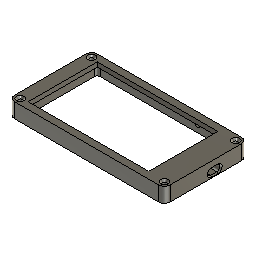
inky-ical (Autodesk Fusion 360 design; units mm, degrees)
Autodesk Fusion 360 part; units mm, degrees
note: some values were not read from the file. Set by a fixed rule: which face or edge a step refers to.
sketch "base" plane through (0, 0, 0) normal (0, 0, 1) x (1, 0, 0)
  line L0 (-5, 62.75) -> (-5, 0)
  line L1 (0, -5) -> (126.75, -5)
  line L2 (0, 67.75) -> (126.75, 67.75)
  line L3 (131.75, 62.75) -> (131.75, 0)
  arc A0 (0, 67.75) -> (-5, 62.75) centre (0, 62.75) ccw
  arc A1 (131.75, 62.75) -> (126.75, 67.75) centre (126.75, 62.75) ccw
  arc A2 (126.75, -5) -> (131.75, 0) centre (126.75, 0) ccw
  arc A3 (-5, 0) -> (0, -5) centre (0, 0) ccw
  line L4 (8, 59.75) -> (110, 59.75)
  line L5 (110, 59.75) -> (110, 3)
  line L6 (110, 3) -> (8, 3)
  line L7 (8, 3) -> (8, 59.75)
  line L8 (3, 64.75) -> (123.75, 64.75)
  line L9 (123.75, 64.75) -> (123.75, -2)
  line L10 (123.75, -2) -> (3, -2)
  line L11 (3, -2) -> (3, 64.75)
  line L12 (3, -2) -> (8, 3) construction
  line L13 (3, 64.75) -> (8, 59.75) construction
  circle A4 centre (0, 62.75) radius 1.75
  circle A5 centre (0, 0) radius 1.75
  circle A6 centre (126.75, 0) radius 1.75
  circle A7 centre (126.75, 62.75) radius 1.75
  dimension "outerCornerRadius" = 5
  dimension "d2" = 5
  dimension "d3" = 5
  dimension "d4" = 5
  dimension "d5" = 102
  dimension "d6" = 56.75
  dimension "d7" = 120.75
  dimension "d8" = 66.75
  dimension "d10" = 3
  dimension "d11" = 3
  dimension "m3ScrewHole" = 3.5
  dimension "d14" = 3.5
  dimension "d15" = 3.5
  dimension "d16" = 3.5
  dimension "d18" = 3
  dimension "d19" = 3
  dimension "d40" = 5
  constraint vertical L0
  constraint horizontal L1
  constraint horizontal L2
  constraint vertical L3
  constraint tangent L0 A0
  constraint tangent L2 A1
  constraint tangent L1 A2
  constraint tangent L1 A3
  constraint tangent L2 A0
  constraint tangent L3 A1
  constraint tangent L3 A2
  constraint tangent L0 A3
  constraint horizontal L4
  constraint vertical L5
  constraint horizontal L6
  constraint vertical L7
  constraint coincident A3.centre A5.centre
  constraint horizontal L8
  constraint vertical L9
  constraint horizontal L10
  constraint vertical L11
  constraint equal L12 L13
  constraint concentric A0 A4
  constraint concentric A2 A6
  constraint concentric A1 A7
  measures "outerCornerRadius" radius of A3
  measures "d2" radius of A0
  measures "d3" radius of A1
  measures "d4" radius of A2
  measures "d5" distance of L5.end L6.end
  measures "d6" distance of L4.end L5.end
  measures "d7" distance of L9.end L10.end
  measures "d8" distance of L8.end L9.end
  measures "d10" distance of L1 L10
  measures "d11" distance of L2 L8
  measures "m3ScrewHole" diameter of A4
  measures "d14" diameter of A5
  measures "d15" diameter of A6
  measures "d16" diameter of A7
  measures "d18" distance of L11 A0.centre
  measures "d19" distance of A1.centre L9
  measures "d40" distance of L7 L11
  measures "d45" diameter of L3.end
  measures "d53" distance of L3.end
  measures "d59" diameter of L3.end
  measures "d60" diameter of L3.end
extrude "Extrude1" add sketch "base" along normal blind 13 contours L0 L1 L2 L3 A0 A1 A2 A3 | L8 L9 L10 L11 makes body 1
chamfer "Chamfer1" distance 1.6 angle 45 4 edges at (-1.6316, 0.6328, 13) (-1.6316, 63.3828, 13) (125.1184, 63.3828, 13) (125.1184, 0.6328, 13) tangent chain off on bodies 1
extrude "Extrude2" cut sketch "base" along normal blind 11 contours L8 L9 L10 L11 bodies 1
chamfer "Chamfer3" distance 2 angle 45 4 edges at (59, 3, 13) (110, 31.375, 13) (8, 31.375, 13) (59, 59.75, 13) tangent chain off on bodies 1
extrude "Extrude3" add sketch "base" against normal blind 8.5 separate body contours L0 L1 L2 L3 A0 A1 A2 A3 | L4 L5 L6 L7 | L8 L9 L10 L11 | A4 | A5 | A6 | A7 makes body 2
sketch "battery-magnet-recess" plane through (0, 0, 0) normal (0, 0, 1) x (-1, 0, 0)
  arc A0 (0, -67.75) -> (5, -62.75) centre (0, -62.75) ccw
  line L0 (5, -62.75) -> (5, 0)
  arc A1 (5, 0) -> (0, 5) centre (0, 0) ccw
  line L1 (0, 5) -> (-126.75, 5)
  arc A2 (-126.75, 5) -> (-131.75, 0) centre (-126.75, 0) ccw
  line L2 (-131.75, 0) -> (-131.75, -62.75)
  arc A3 (-131.75, -62.75) -> (-126.75, -67.75) centre (-126.75, -62.75) ccw
  line L3 (-126.75, -67.75) -> (0, -67.75)
  line L4 (-109.75, -0.875) -> (-15.75, -0.875)
  line L5 (-15.75, -0.875) -> (-15.75, -61.875)
  line L6 (-15.75, -61.875) -> (-109.75, -61.875)
  line L7 (-109.75, -61.875) -> (-109.75, -0.875)
  line L8 (-3, 2) -> (-3, -64.75)
  line L9 (-123.75, 2) -> (-3, 2)
  circle A4 centre (-126.75, 0) radius 2.25
  circle A5 centre (-126.75, -62.75) radius 2.25
  circle A6 centre (0, -62.75) radius 2.25
  circle A7 centre (0, 0) radius 2.25
  line L10 (-109.75, -31.375) -> (-131.75, -31.375) construction
  circle A8 centre (-3, -9.375) radius 4.1
  circle A9 centre (-3, -53.375) radius 4.1
  circle A10 centre (-123.75, -53.375) radius 4.1
  circle A11 centre (-123.75, -9.375) radius 4.1
  line L11 (-3, -53.375) -> (-3, -9.375) construction
  line L12 (-123.75, -53.375) -> (-123.75, -9.375) construction
  line L13 (5, -31.375) -> (-3, -31.375) construction
  line L14 (-123.75, -31.375) -> (-131.75, -31.375) construction
  dimension "d29" = 61
  dimension "d30" = 94
  dimension "d33" = 4.5
  dimension "d53" = 22
  dimension "d57" = 8.2
  dimension "d58" = 8.2
  dimension "d59" = 8.2
  dimension "d60" = 8.2
  dimension "d64" = 8
  dimension "d65" = 44
  dimension "d66" = 8
  constraint horizontal L4
  constraint vertical L5
  constraint horizontal L6
  constraint vertical L7
  constraint concentric A2 A4
  constraint concentric A3 A5
  constraint concentric A0 A6
  constraint concentric A1 A7
  constraint equal A4 A7
  constraint equal A4 A6
  constraint equal A4 A5
  constraint coincident L7 L10.start
  constraint coincident L2 L10.end
  constraint perpendicular L2 L10
  constraint midpoint L2 L10.end
  constraint midpoint L7 L10.start
  constraint coincident A9.centre L11.start
  constraint coincident A8.centre L11.end
  constraint coincident A10.centre L12.start
  constraint coincident A11.centre L12.end
  constraint vertical L11
  constraint vertical L12
  constraint coincident L0 L13.start
  constraint coincident L11 L13.end
  constraint perpendicular L11 L13
  constraint midpoint L11 L13.end
  constraint midpoint L0 L13.start
  constraint equal L11 L12
  constraint coincident L12 L14.start
  constraint perpendicular L2 L14
  constraint midpoint L12 L14.start
  measures "d29" distance of L4.start L6.end
  measures "d30" distance of L5.end L6.end
  measures "d33" diameter of A4
  measures "d53" distance of L10.start L10.end
  measures "d57" diameter of A8
  measures "d58" diameter of A9
  measures "d59" diameter of A10
  measures "d60" diameter of A11
  measures "d64" distance of L13.start L13.end
  measures "d65" distance of A9.centre A8.centre
  measures "d66" distance of L14.start L10.end
extrude "Extrude4" cut sketch "battery-magnet-recess" against normal blind 6.5 contours L4 L5 L6 L7 bodies 2
extrude "Extrude5" cut sketch "battery-magnet-recess" against normal blind 19 contours A4 | A5 | A6 | A7 bodies 2
fillet "Fillet1" radius 2.5 4 edges at (123.75, 64.75, 5.5) (3, 64.75, 5.5) (3, -2, 5.5) (123.75, -2, 5.5) on bodies 1
fillet "Fillet2" radius 3 2 edges at (62.75, 61.875, -6.5) (62.75, 0.875, -6.5) on bodies 2
sketch "usb-hole" plane through (131.75, 0, 0) normal (1, 0, 0) x (0, 1, 0)
  line L0 (0, 0) -> (62.75, 0)
  line L1 (62.75, 0) -> (62.75, 13)
  line L2 (62.75, 13) -> (0, 13)
  line L3 (0, 13) -> (0, 0)
  line L4 (42, 1.5) -> (36.5, 1.5)
  line L5 (42, 7) -> (36.5, 7)
  arc A0 (42, 1.5) -> (42, 7) centre (42, 4.25) ccw
  arc A1 (36.5, 7) -> (36.5, 1.5) centre (36.5, 4.25) ccw
  line L6 (33.75, 2.1871) -> (33.75, 6.5143) construction
  line L7 (44.75, 2.1572) -> (44.75, 6.4585) construction
  line L8 (62.75, 0) -> (0, 0) construction
  dimension "d41" = 5.5
  dimension "d42" = 11
  dimension "d43" = 1.5
  dimension "d44" = 18
  constraint parallel L2 L4
  constraint parallel L2 L5
  constraint tangent L4 A0
  constraint tangent L4 A1
  constraint equal L4 L5
  constraint tangent L5 A0
  constraint vertical L7
  constraint vertical L6
  constraint tangent A0 L7
  constraint tangent A1 L6
  measures "d41" distance of L4 L5
  measures "d42" distance of L6 L7
  measures "d43" distance of L4 L8
  measures "d44" distance of L1 L7
sketch "reset-button-hole" plane through (0, 67.75, 0) normal (0, 1, 0) x (-1, 0, 0)
  line L0 (-126.75, 0) -> (0, 0)
  line L1 (0, 0) -> (0, 13)
  line L2 (0, 13) -> (-126.75, 13)
  line L3 (-126.75, 13) -> (-126.75, 0)
  circle A0 centre (-91.25, 6.75) radius 2.5
  line L4 (0, 0) -> (-126.75, 0)
  dimension "d45" = 5
  dimension "d46" = 6.75
  dimension "d47" = 35.5
  measures "d45" diameter of A0
  measures "d46" distance of A0.centre L4
  measures "d47" distance of L3 A0.centre
extrude "Extrude6" cut sketch "usb-hole" against normal blind 12 contours L4 L5 A0 A1 bodies 1
extrude "Extrude7" cut sketch "reset-button-hole" against normal blind 7 contours A0 bodies 1
extrude "Extrude9" cut sketch "battery-magnet-recess" against normal blind 8.125 contours L8 A8 | L8 A8 | L8 A9 | L8 A9 | A10 | A11 bodies 2
sketch "mounting-pillars" plane through (0, 0, 0) normal (0, 0, 1) x (-1, 0, 0)
  circle A0 centre (-126.75, 0) radius 2.25
  circle A1 centre (0, 0) radius 2.25
  circle A2 centre (-126.75, -62.75) radius 2.25
  circle A3 centre (0, -62.75) radius 2.25
  arc A4 (0, -67.75) -> (5, -62.75) centre (0, -62.75) ccw
  line L0 (5, -62.75) -> (5, 0)
  arc A5 (5, 0) -> (0, 5) centre (0, 0) ccw
  line L1 (0, 5) -> (-126.75, 5)
  arc A6 (-126.75, 5) -> (-131.75, 0) centre (-126.75, 0) ccw
  line L2 (-131.75, 0) -> (-131.75, -62.75)
  arc A7 (-131.75, -62.75) -> (-126.75, -67.75) centre (-126.75, -62.75) ccw
  line L3 (-126.75, -67.75) -> (0, -67.75)
  line L4 (-109.75, -61.875) -> (-109.75, -0.875)
  line L5 (-109.75, -0.875) -> (-15.75, -0.875)
  line L6 (-15.75, -0.875) -> (-15.75, -61.875)
  line L7 (-15.75, -61.875) -> (-109.75, -61.875)
  circle A8 centre (-123.75, -9.375) radius 4.1
  circle A9 centre (-3, -53.375) radius 4.1
  circle A10 centre (-123.75, -53.375) radius 4.1
  circle A11 centre (-3, -9.375) radius 4.1
  circle A12 centre (-8.5, -15.25) radius 1.75
  line L8 (-8.5, -15.25) -> (-8.5, -58.75) construction
  circle A13 centre (-8.5, -58.75) radius 1.75
  circle A14 centre (-117, -4.75) radius 1.75
  line L9 (-117, -4.75) -> (-117, -58.75) construction
  circle A15 centre (-117, -58.75) radius 1.75
  line L10 (-8.5, -58.75) -> (-117, -58.75) construction
  dimension "d69" = 13.5
  dimension "d71" = 3.5
  dimension "d72" = 43.5
  dimension "d73" = 14.75
  dimension "d74" = 54
  dimension "d78" = 9
  constraint coincident A12.centre L8.start
  constraint vertical L8
  constraint coincident L8.end A13.centre
  constraint equal A12 A13
  constraint coincident A14.centre L9.start
  constraint equal A12 A14
  constraint vertical L9
  constraint coincident L9.end A15.centre
  constraint equal A14 A15
  constraint horizontal L10
  measures "d69" distance of L0 A12.centre
  measures "d71" diameter of A12
  measures "d72" distance of A12.centre L8.end
  measures "d73" distance of L2 A14.centre
  measures "d74" distance of A14.centre L9.end
  measures "d78" distance of L3 L8.end
extrude "Extrude10" add sketch "mounting-pillars" along normal blind 8.75 contours A12 | A13 | A14 | A15 bodies 2
sketch "mounting-pillars-notch" plane through (0, 0, 8.75) normal (0, 0, 1) x (-1, 0, 0)
  line L0 (-113.5, -63.25) -> (-116.5, -63.25)
  line L1 (-116.5, -63.25) -> (-116.5, -1.25)
  line L2 (-116.5, -1.25) -> (-113.5, -1.25)
  line L3 (-113.5, -1.25) -> (-113.5, -63.25)
  circle A0 centre (-117, -58.75) radius 1.75
  circle A1 centre (-117, -4.75) radius 1.75
  circle A2 centre (-8.5, -15.25) radius 1.75
  circle A3 centre (-8.5, -58.75) radius 1.75
  dimension "d81" = 62
  dimension "d82" = 3
  constraint horizontal L0
  constraint vertical L1
  constraint horizontal L2
  constraint vertical L3
  measures "d81" distance of L0.start L2.end
  measures "d82" distance of L1.end L2.end
extrude "Extrude11" cut sketch "mounting-pillars-notch" against normal blind 2 contours L0 L1 L2 L3 A0 A1 | L1 A0 | L1 A1 picked at (-115.9308, -58.2791) picked at (-115.8812, -4.3456) bodies 2
move_face "OffsetFaces1" offset 1 2 faces at (117.1847, 58.1923, 8.75) (117.905, 4.2481, 8.75) on bodies 2
chamfer "Chamfer5" distance 1 angle 45 4 edges at (131.75, 39.25, 7) (131.75, 44.75, 4.25) (131.75, 39.25, 1.5) (131.75, 33.75, 4.25) tangent chain off on bodies 1
hidden bodies 2
equation "d2 = outerCornerRadius"
equation "d3 = outerCornerRadius"
equation "d4 = outerCornerRadius"
equation "d14 = m3ScrewHole"
equation "d15 = m3ScrewHole"
equation "d16 = m3ScrewHole"
equation "m3ScrewChamfer = 1.6 mm"
equation "magnetSize = 8.2 mm"
equation "d57 = magnetSize"
equation "d58 = magnetSize"
equation "d59 = magnetSize"
equation "d60 = magnetSize"
named bodies: "inky-ical-front", "inky-ical-rear"
